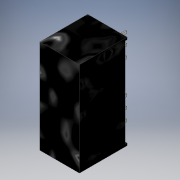
# Autodesk Inventor part: Converter_DCDC_XP_POWER-ITQxxxx-H_SIP_THT
Saved by Autodesk Inventor 2019.1 (Build 231200000, 200)
## iProperties
Created: 2018-08-28
Part Number: Converter_DCDC_XP_POWER-ITQxxxx-H_SIP_THT
Material: Generic
Document SubType Name: Modeling
Designer: huesof
Density: 1 g/cm^3
Appearance: Default
Author: huesof
Autodesk Inventor part; units mm, degrees
ref_plane "YZ Plane" through (0, 0, 0) normal (1, 0, 0) x (0, 1, 0)
ref_plane "XZ Plane" through (0, 0, 0) normal (0, 1, 0) x (-1, 0, 0)
ref_plane "XY Plane" through (0, 0, 0) normal (0, 0, 1) x (1, 0, 0)
sketch "Sketch2" plane through (0, 0, 0) normal (0, 0, 1) x (1, 0, 0)
  line L0 (-6, 2.035) -> (3.2, 2.035)
  line L1 (3.2, 2.035) -> (3.2, -19.815)
  line L2 (3.2, -19.815) -> (-6, -19.815)
  line L3 (-6, -19.815) -> (-6, 2.035)
  line L4 (-0.125, -0.25) -> (0.125, -0.25)
  line L5 (0.125, -0.25) -> (0.125, 0.25)
  line L6 (0.125, 0.25) -> (-0.125, 0.25)
  line L7 (-0.125, 0.25) -> (-0.125, -0.25)
  line L8 (-0.125, -0.25) -> (0.125, 0.25) construction
  line L9 (0.125, -0.25) -> (-0.125, 0.25) construction
  line L10 (-0.125, -2.79) -> (0.125, -2.79)
  line L11 (0.125, -2.79) -> (0.125, -2.29)
  line L12 (0.125, -2.29) -> (-0.125, -2.29)
  line L13 (-0.125, -2.29) -> (-0.125, -2.79)
  line L14 (-0.125, -2.79) -> (0.125, -2.29) construction
  line L15 (0.125, -2.79) -> (-0.125, -2.29) construction
  line L16 (-0.125, -12.45) -> (0.125, -12.45)
  line L17 (0.125, -12.45) -> (0.125, -12.95)
  line L18 (0.125, -12.95) -> (-0.125, -12.95)
  line L19 (-0.125, -12.95) -> (-0.125, -12.45)
  line L20 (-0.125, -12.45) -> (0.125, -12.95) construction
  line L21 (0.125, -12.45) -> (-0.125, -12.95) construction
  line L22 (-0.125, -14.99) -> (0.125, -14.99)
  line L23 (0.125, -14.99) -> (0.125, -15.49)
  line L24 (-0.125, -15.49) -> (-0.125, -14.99)
  line L25 (-0.125, -14.99) -> (0.125, -15.49) construction
  line L26 (0.125, -14.99) -> (-0.125, -15.49) construction
  line L27 (0.125, -15.49) -> (-0.125, -15.49)
  line L28 (-0.125, -17.53) -> (0.125, -17.53)
  line L29 (0.125, -17.53) -> (0.125, -18.03)
  line L30 (-0.125, -18.03) -> (-0.125, -17.53)
  line L31 (-0.125, -17.53) -> (0.125, -18.03) construction
  line L32 (0.125, -17.53) -> (-0.125, -18.03) construction
  line L33 (0.125, -18.03) -> (-0.125, -18.03)
  line L34 (-6, 2.035) -> (3.2, 2.035)
  line L35 (3.2, 2.035) -> (3.2, 1.535)
  line L36 (3.2, 1.535) -> (-6, 1.535)
  line L37 (-6, 1.535) -> (-6, 2.035)
  line L38 (-6, -19.815) -> (3.2, -19.815)
  line L39 (3.2, -19.815) -> (3.2, -19.315)
  line L40 (3.2, -19.315) -> (-6, -19.315)
  line L41 (-6, -19.315) -> (-6, -19.815)
  line L42 (-0.125, -5.33) -> (0.125, -5.33)
  line L43 (0.125, -5.33) -> (0.125, -4.83)
  line L44 (0.125, -4.83) -> (-0.125, -4.83)
  line L45 (-0.125, -4.83) -> (-0.125, -5.33)
  line L46 (-0.125, -5.33) -> (0.125, -4.83) construction
  line L47 (0.125, -5.33) -> (-0.125, -4.83) construction
  point P0 (0, 0)
  point P1 (0, -2.54)
  point P2 (0, -12.7)
  point P3 (0, -15.24)
  point P4 (0, -17.78)
  point P5 (0, -5.08)
  dimension "d37" = 2.035
  dimension "d38" = 3.2
  dimension "d40" = 9.2
  dimension "d41" = 0.25
  dimension "d42" = 0.5
  dimension "d45" = 2.54
  dimension "d50" = 0.25
  dimension "d51" = 0.5
  dimension "d52" = 0
  dimension "d53" = 12.7
  dimension "d56" = 2.54
  dimension "d61" = 0.5
  dimension "d62" = 0.5
  dimension "d72" = 21.85
  constraints: 96 end point, 12 midpoint, 10 parallel, 5 horizontal, 5 perpendicular, 2 point on line, 2 vertical, 1 collinear, 43 other
  measures "d37" distance from line of L0 point (0, 0)
  measures "d38" distance from line of point (0, 0) L1
  measures "d40" distance between parallel lines of L1 L3
  measures "d41" distance of L6.end L5.end
  measures "d42" distance of L5.end L4.end
  measures "d45" distance of L4.start L10.start
  measures "d50" distance of L16.start L16.end
  measures "d51" distance of L16.end L17.end
  measures "d52" horizontal distance of point (0, 0) point (0, -12.7)
  measures "d53" distance of point (0, 0) point (0, -12.7)
  measures "d56" distance of L16.start L22.start
  measures "d61" distance of L34.end L35.end
  measures "d62" distance of L39.end L38.end
  measures "d72" distance between parallel lines of L2 L0
extrude "Extrusion4" add sketch "Sketch2" along normal blind 10.6 contours L0 L1 L36 L3 | L36 L1 L40 L3 | L40 L1 L2 L3 | L7 L6 L5 L4 | L13 L12 L11 L10 | L16 L17 L18 L19 | L22 L23 L27 L24 | L28 L29 L33 L30 | L45 L44 L43 L42
extrude "Extrusion5" add sketch "Sketch2" against normal blind 0.5 contours L0 L1 L36 L3 | L40 L1 L2 L3
extrude "Extrusion6" add sketch "Sketch2" against normal blind 3.5 separate body contours L7 L6 L5 L4 | L13 L12 L11 L10 | L16 L17 L18 L19 | L22 L23 L27 L24 | L28 L29 L33 L30 | L45 L44 L43 L42
move or copy body "Move Body1" bodies to move or copy 1 2 copy no translate (0, 0, 0.5)
equation "\"d50\" = d41"
equation "\"d51\" = d42"
body "Solid1"
body "Solid3"
body "Solid4"
